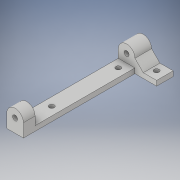
# Autodesk Inventor part: 000.208 - Рама крышки портов Raspberry
Saved by Autodesk Inventor 2019 (Build 230136000, 136)
## iProperties
Created: 2020-03-06
Part Number: 000.208 - Рама крышки портов Raspberry
Material: Типовые
Document SubType Name: Modeling
Designer: Петров Иван
Density: 1 g/cm^3
Appearance: По умолчанию
Author: Петров Иван
Autodesk Inventor part; units mm, degrees
ref_plane "YZ Plane" through (0, 0, 0) normal (1, 0, 0) x (0, 1, 0)
ref_plane "XZ Plane" through (0, 0, 0) normal (0, 1, 0) x (-1, 0, 0)
ref_plane "XY Plane" through (0, 0, 0) normal (0, 0, 1) x (1, 0, 0)
sketch "Эскиз1" plane through (0, 0, 0) normal (0, 1, 0) x (-1, 0, 0)
  line L0 (-6.5, 30) -> (6.5, 30)
  line L1 (6.5, 30) -> (6.5, -30)
  line L2 (6.5, -30) -> (-6.5, -30)
  line L3 (-6.5, -30) -> (-6.5, 30)
  line L4 (-6.5, 30) -> (6.5, -30) construction
  line L5 (6.5, 30) -> (-6.5, -30) construction
  line L6 (6.5, 30) -> (16.5, 30)
  line L7 (16.5, 30) -> (16.5, -30)
  line L8 (16.5, -30) -> (6.5, -30)
  line L9 (6.5, -30) -> (6.5, 30)
  line L10 (16.5, -30) -> (-6.5, -30)
  line L11 (-6.5, -30) -> (-6.5, -40)
  line L12 (-6.5, -40) -> (16.5, -40)
  line L13 (16.5, -40) -> (16.5, -30)
  point P0 (0, 0)
  dimension "d0" = 13
  dimension "d1" = 60
  dimension "d2" = 10
  dimension "d3" = 60
  dimension "d4" = 23
  dimension "d5" = 10
  constraints: 28 end point, 6 parallel, 3 horizontal, 3 perpendicular, 2 midpoint
  measures "d0" distance of L1.end L2.end
  measures "d1" distance of L0.end L1.end
  measures "d2" distance of L7.end L8.end
  measures "d3" distance of L6.end L7.end
  measures "d4" distance of L12.end L11.end
  measures "d5" distance of L11.end L10.end
extrude "Выдавливание1" add sketch "Эскиз1" along normal blind 3 contours L6 L7 L8 L1 | L2 L8 L13 L12 L11
sketch "Эскиз2" plane through (0, 3, 0) normal (0, 1, 0) x (1, 0, 0)
  line L0 (-6.5, -30) -> (-6.5, 30) projected
  line L1 (6.5, 40) -> (-16.5, 40) projected
  line L2 (-6.5, 30) -> (-16.5, 30)
  line L3 (-16.5, 30) -> (-16.5, 40)
  line L4 (-16.5, 40) -> (-6.5, 40)
  line L5 (-6.5, 40) -> (-6.5, 30)
  point P0 (0, 0)
  constraints: 8 end point, 2 parallel, 1 horizontal, 1 perpendicular
extrude "Выдавливание2" add sketch "Эскиз2" along normal blind 10
sketch "Эскиз3" plane through (-16.5, 3, -30) normal (0, 0, 1) x (1, 0, 0)
  line L0 (10, 0) -> (10, 10) projected
  line L1 (10, 5) -> (0, 5)
  line L2 (0, -3) -> (0, 10) projected
  circle A0 centre (5, 5) radius 1.5
  point P0 (16.5, -3)
  dimension "d10" = 3
  constraints: 2 end point, 2 midpoint, 1 centre point, 1 horizontal, 1 point on line
  measures "d10" diameter of A0
extrude "Выдавливание3" cut sketch "Эскиз3" against normal blind 10
fillet "Сопряжение1" radius 5 2 edges at (-6.5, 13, -35) (-16.5, 13, -35)
chamfer "Фаска1" distance 5 angle 45 1 edges at (-6.5, 3, -35)
sketch "Эскиз4" plane through (0, 3, 0) normal (0, 1, 0) x (1, 0, 0)
  line L0 (-16.5, -30) -> (-6.5, -30) projected
  line L1 (-11.5, -30) -> (-11.5, -15)
  circle A0 centre (-11.5, -15) radius 1.5
  line L2 (6.5, 30) -> (6.5, 40) projected
  line L3 (6.5, 35) -> (1.5, 35)
  circle A1 centre (1.5, 35) radius 1.5
  circle A2 centre (-11.5, 25) radius 1.5
  line L4 (-16.5, 40) -> (-6.5, 40) projected
  point P0 (0, 0)
  dimension "d17" = 15
  dimension "d18" = 3
  dimension "d19" = 5
  dimension "d20" = 3
  dimension "d21" = 3
  dimension "d22" = 15
  constraints: 4 end point, 3 centre point, 2 coincident, 2 midpoint, 1 horizontal, 1 vertical
  measures "d17" distance of L1.start L1.end
  measures "d18" diameter of A0
  measures "d19" distance of L3.start L3.end
  measures "d20" diameter of A1
  measures "d21" diameter of A2
  measures "d22" distance from line of L4 A2.centre
extrude "Выдавливание4" cut sketch "Эскиз4" against normal through all
sketch "Эскиз5" plane through (0, 3, 0) normal (0, 1, 0) x (1, 0, 0)
  line L0 (-16.5, -30) -> (-6.5, -30) projected
  line L1 (-16.5, -30) -> (-6.5, -30)
  line L2 (-6.5, -30) -> (-6.5, -37)
  line L3 (-6.5, -37) -> (-16.5, -37)
  line L4 (-16.5, -37) -> (-16.5, -30)
  point P0 (0, 0)
  dimension "d25" = 7
  constraints: 8 end point, 2 parallel, 1 horizontal, 1 perpendicular
  measures "d25" distance of L1.end L2.end
extrude "Выдавливание5" add sketch "Эскиз5" along normal blind 10 and the other way blind 3
sketch "Эскиз6" plane through (-16.5, 13, 37) normal (0, 0, 1) x (1, 0, 0)
  circle A0 centre (5, -5) radius 1.5 projected
  arc A1 (10, -5) -> (0, -5) centre (5, -5) ccw projected
  line L0 (0, 0) -> (0, -13) projected
  line L1 (0, 0) -> (10, 0) projected
  line L2 (10, 0) -> (10, -13) projected
  point P0 (16.5, -13)
extrude "Выдавливание6" cut sketch "Эскиз6" against normal blind 10 contours A0
fillet "Сопряжение2" radius 5 2 edges at (-6.5, 13, 33.5) (-16.5, 13, 33.5)
